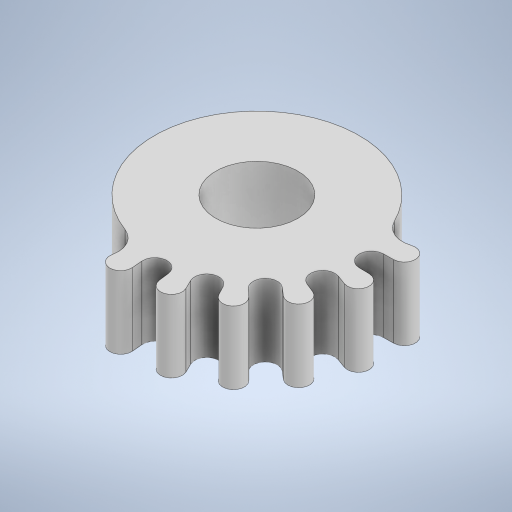
# Autodesk Inventor part: End_Effector_Claw_L_test
Saved by Autodesk Inventor 2023 (Build 270158000, 158)
## iProperties
Created: 2025-02-27
Part Number: End_Effector_Claw_L_test
Material: Generic
Document SubType Name: Modeling
Designer: Swoby
Density: 1 g/cm^3
Appearance: Default
Author: Swoby
Autodesk Inventor part; units mm, degrees
ref_plane "YZ Plane" through (0, 0, 0) normal (1, 0, 0) x (0, 1, 0)
ref_plane "XZ Plane" through (0, 0, 0) normal (0, 1, 0) x (-1, 0, 0)
ref_plane "XY Plane" through (0, 0, 0) normal (0, 0, 1) x (1, 0, 0)
sketch "Sketch1" plane through (0, 0, 0) normal (0, 1, 0) x (-1, 0, 0)
  line L0 (0, 0) -> (10, 0) construction
  circle A0 centre (10, 0) radius 8.5
  line L1 (0, 0) -> (-10, 0) construction
  circle A1 centre (-10, 0) radius 8.5 construction
  line L2 (10, 0) -> (21.547, -20) construction
  line L3 (21.547, -20) -> (21.547, -40) construction
  line L4 (21.547, -40) -> (0, -65.6787) construction
  line L5 (0, -69.6065) -> (0, -61.751)
  arc A2 (0, -61.751) -> (5.0646, -19.2801) centre (-15.4138, -38.3755) ccw
  line L6 (15.5832, -6.4092) -> (26.547, -19.4754) construction
  line L7 (26.547, -19.4754) -> (26.547, -49.4754)
  line L8 (26.547, -49.4754) -> (1.6428, -70.3725)
  arc A3 (4.4168, -6.4092) -> (5.0646, -19.2801) centre (12.3783, -12.4603) ccw
  arc A4 (5.0646, -19.2801) -> (0, -15) centre (-15.4138, -38.3755) ccw construction
  line L9 (15.5832, -6.4092) -> (4.4168, -6.4092) construction
  arc A5 (18.4809, 0.5693) -> (26.547, -19.4754) centre (53.2139, 2.9008) ccw
  arc A6 (0, -69.6065) -> (1.6428, -70.3725) centre (1, -69.6065) ccw
  circle A7 centre (10, 0) radius 1.75
  circle A8 centre (10, 0) radius 3.4
  point P0 (0, -71.751)
  dimension "d0" = 10
  dimension "d1" = 17
  dimension "d2" = 10
  dimension "d3" = 17
  dimension "d4" = 120
  dimension "d5" = 140
  dimension "d6" = 20
  dimension "d9" = 20
  dimension "d10" = 65.6787
  dimension "d11" = 10
  dimension "d12" = 15
  dimension "d14" = 50
  dimension "d15" = 5
  dimension "d16" = 30
  dimension "d18" = 10
  dimension "d19" = 28
  dimension "d20" = 1
  dimension "d52" = 3.5
  dimension "d53" = 6.8
  constraints: 20 end point, 13 point on circle, 9 centre point, 5 tangent, 4 coincident, 4 point on line, 3 horizontal, 3 vertical, 1 midpoint, 1 perpendicular
  measures "d0" distance of L0.start L0.end
  measures "d1" diameter of A0
  measures "d2" distance of L0.start L1.end
  measures "d3" diameter of A1
  measures "d4" angle of L0 L2
  measures "d5" angle of L3 L4
  measures "d6" distance of L2.end L3.end
  measures "d9" vertical distance of L2.start L2.end
  measures "d10" vertical distance of L4.end L0.end
  measures "d11" distance of point (0, -71.751) L5.end
  measures "d12" distance of L0.start A4.end
  measures "d14" angle of L6 L0
  measures "d15" distance between parallel lines of L3 L7
  measures "d16" distance of L6.end L7.end
  measures "d18" radius of A3
  measures "d19" radius of A2
  measures "d20" radius of A6
  measures "d52" diameter of A7
  measures "d53" diameter of A8
extrude "Extrusion1" add sketch "Sketch1" along normal blind 4 contours A0 | A0 A5 L7 L8 A6 L5 A2 A3 | A8
sketch "Sketch2" plane through (0, 4, 0) normal (0, 1, 0) x (1, 0, 0)
  arc A0 (-18.4809, -0.5693) -> (-4.4168, 6.4092) centre (-10, 0) ccw projected
  circle A1 centre (10, 0) radius 8.5 construction
  line L0 (10, 0) -> (18.5, 0) construction
  arc A2 (0.3386, 1.0136) -> (1.2091, 2.0775) centre (0.3242, 1.9135) ccw
  arc A3 (-0.5608, -1.7495) -> (1.2091, -2.0775) centre (0.3242, -1.9135) ccw construction
  circle A4 centre (-0.5, 0) radius 0.9 construction
  line L1 (-10, 0) -> (-18.5, 0) construction
  line L2 (-10, 0) -> (0.3242, 1.9135) construction
  line L3 (-10, 0) -> (0.3242, -1.9135) construction
  arc A5 (-0.516, 0.9999) -> (-0.516, -0.9999) centre (-0.5, 0) ccw
  line L4 (-0.516, 0.9999) -> (0.3386, 1.0136)
  line L5 (-0.516, -0.9999) -> (0.3386, -1.0136)
  arc A6 (-0.5608, 1.7495) -> (0.3386, 1.0136) centre (0.3242, 1.9135) ccw construction
  arc A7 (1.2091, 2.0775) -> (0.0395, 2.7673) centre (0.3242, 1.9135) ccw
  arc A8 (0.3386, -1.0136) -> (-0.5608, -1.7495) centre (0.3242, -1.9135) ccw construction
  arc A9 (1.2091, -2.0775) -> (0.3386, -1.0136) centre (0.3242, -1.9135) ccw
  arc A10 (0.0395, 2.7673) -> (-0.5608, 1.7495) centre (0.3242, 1.9135) ccw construction
  arc A11 (-2.3848, 3.7761) -> (0.0395, 2.7673) centre (-0.593, 4.6646) ccw
  arc A12 (-0.2799, -5.9565) -> (-0.7113, -4.6513) centre (-1.0473, -5.4862) ccw
  line L6 (-1.5043, -4.3322) -> (-0.7113, -4.6513)
  arc A13 (-0.7876, -2.4653) -> (-1.5043, -4.3322) centre (-1.131, -3.4045) ccw
  line L7 (-0.7876, -2.4653) -> (0.0152, -2.7588)
  arc A14 (0.0152, -2.7588) -> (1.2091, -2.0775) centre (0.3242, -1.9135) ccw
  arc A15 (-3.0601, -9.0442) -> (-2.9951, -7.6711) centre (-3.608, -8.3302) ccw
  line L8 (-3.6211, -7.0891) -> (-2.9951, -7.6711)
  arc A16 (-2.283, -5.603) -> (-3.6211, -7.0891) centre (-2.9401, -6.3567) ccw
  line L9 (-2.283, -5.603) -> (-1.6387, -6.1646)
  arc A17 (-1.6387, -6.1646) -> (-0.2799, -5.9565) centre (-1.0473, -5.4862) ccw
  arc A18 (-6.7622, -10.9305) -> (-6.2095, -9.6719) centre (-7.0178, -10.0676) ccw
  line L10 (-6.5853, -8.9042) -> (-6.2095, -9.6719)
  arc A19 (-4.8035, -7.9963) -> (-6.5853, -8.9042) centre (-5.6871, -8.4646) ccw
  line L11 (-4.8035, -7.9963) -> (-4.4033, -8.7516)
  arc A20 (-4.4033, -8.7516) -> (-3.0601, -9.0442) centre (-3.608, -8.3302) ccw
  arc A21 (-10.8944, -11.3649) -> (-9.9274, -10.3879) centre (-10.8238, -10.4676) ccw
  line L12 (-10.0031, -9.5365) -> (-9.9274, -10.3879)
  arc A22 (-8.0143, -9.3275) -> (-10.0031, -9.5365) centre (-9.007, -9.448) ccw
  line L13 (-8.0143, -9.3275) -> (-7.9113, -10.176)
  arc A23 (-7.9113, -10.176) -> (-6.7622, -10.9305) centre (-7.0178, -10.0676) ccw
  arc A24 (-11.7027, -10.2738) -> (-12.9594, -7.9682) centre (-13.6558, -9.843) ccw
  arc A25 (-11.7027, -10.2738) -> (-10.8944, -11.3649) centre (-10.8238, -10.4676) ccw
  point P0 (0, 0)
  point P1 (-9.1115, -8.4534)
  point P2 (-6.1411, -7.5736)
  point P3 (-3.6833, -5.6876)
  point P4 (-2.0646, -3.0461)
  point P5 (-0.2799, -5.9565)
  point P6 (-1.5, 0)
  dimension "d26" = 17
  dimension "d23" = 10
  dimension "d24" = 10
  dimension "d25" = 8.5
  dimension "d36" = 1.8
  dimension "d37" = 1.8
  dimension "d38" = 1.8
  dimension "d39" = 10.5
  dimension "d40" = 10.5
  dimension "d41" = 21
  dimension "d42" = 10.5
  dimension "d43" = 10.5
  dimension "d44" = 2
  dimension "d47" = 84
  dimension "d49" = 2
  dimension "d58" = 9.5
  constraints: 48 point on circle, 28 end point, 24 centre point, 12 tangent, 6 point on line, 2 horizontal, 1 coincident, 1 concentric, 1 horizontal alignment, 59 other
  measures "d23" distance of L1.start point (0, 0)
  measures "d24" distance of L0.start point (0, 0)
  measures "d25" radius of A0
  measures "d36" diameter of A2
  measures "d37" diameter of A3
  measures "d38" diameter of A4
  measures "d39" distance of L1.start L2.end
  measures "d40" distance of L1.start L3.end
  measures "d41" angle of L3 L2
  measures "d42" angle of L1 L2
  measures "d43" distance of L0.start A4.centre
  measures "d44" radius of A11
  measures "d49" radius of A24
  measures "d58" distance of A4.centre L1.start
extrude "Extrusion2" add sketch "Sketch2" against normal up to surface (4 mm away)
extrude "Extrusion4" cut sketch "Sketch1" against normal blind 1 from surface at 4 contours A8
sketch "Sketch3" plane through (0, 4, 0) normal (0, 1, 0) x (1, 0, 0)
  circle A0 centre (-10, 0) radius 3.4 projected
  arc A1 (-4.4168, 6.4092) -> (-5.0646, 19.2801) centre (-12.3783, 12.4603) ccw projected
  arc A2 (0, 61.751) -> (-5.0646, 19.2801) centre (15.4138, 38.3755) ccw projected
  line L0 (0, 61.751) -> (0, 69.6065) projected
  arc A3 (0, 69.6065) -> (-1.6428, 70.3725) centre (-1, 69.6065) ccw projected
  line L1 (-1.6428, 70.3725) -> (-26.547, 49.4754) projected
  line L2 (-26.547, 49.4754) -> (-26.547, 19.4754) projected
  arc A4 (-18.4809, -0.5693) -> (-26.547, 19.4754) centre (-53.2139, -2.9008) ccw projected
  arc A5 (-18.4809, -0.5693) -> (-12.9594, -7.9682) centre (-10, 0) ccw projected
  arc A6 (-11.7027, -10.2738) -> (-12.9594, -7.9682) centre (-13.6558, -9.843) ccw projected
  arc A7 (-11.7027, -10.2738) -> (-9.9274, -10.3879) centre (-10.8238, -10.4676) ccw projected
  line L3 (-9.9274, -10.3879) -> (-10.0031, -9.5365) projected
  arc A8 (-8.0143, -9.3275) -> (-10.0031, -9.5365) centre (-9.007, -9.448) ccw projected
  line L4 (-8.0143, -9.3275) -> (-7.9113, -10.176) projected
  arc A9 (-7.9113, -10.176) -> (-6.2095, -9.6719) centre (-7.0178, -10.0676) ccw projected
  line L5 (-6.2095, -9.6719) -> (-6.5853, -8.9042) projected
  arc A10 (-4.8035, -7.9963) -> (-6.5853, -8.9042) centre (-5.6871, -8.4646) ccw projected
  line L6 (-4.8035, -7.9963) -> (-4.4033, -8.7516) projected
  arc A11 (-4.4033, -8.7516) -> (-2.9951, -7.6711) centre (-3.608, -8.3302) ccw projected
  line L7 (-2.9951, -7.6711) -> (-3.6211, -7.0891) projected
  arc A12 (-2.283, -5.603) -> (-3.6211, -7.0891) centre (-2.9401, -6.3567) ccw projected
  line L8 (-2.283, -5.603) -> (-1.6387, -6.1646) projected
  arc A13 (-1.6387, -6.1646) -> (-0.7113, -4.6513) centre (-1.0473, -5.4862) ccw projected
  line L9 (-0.7113, -4.6513) -> (-1.5043, -4.3322) projected
  arc A14 (-0.7876, -2.4653) -> (-1.5043, -4.3322) centre (-1.131, -3.4045) ccw projected
  line L10 (-0.7876, -2.4653) -> (0.0152, -2.7588) projected
  arc A15 (0.0152, -2.7588) -> (0.3386, -1.0136) centre (0.3242, -1.9135) ccw projected
  line L11 (0.3386, -1.0136) -> (-0.516, -0.9999) projected
  arc A16 (-0.516, 0.9999) -> (-0.516, -0.9999) centre (-0.5, 0) ccw projected
  line L12 (-0.516, 0.9999) -> (0.3386, 1.0136) projected
  arc A17 (0.3386, 1.0136) -> (0.0395, 2.7673) centre (0.3242, 1.9135) ccw projected
  arc A18 (-2.3848, 3.7761) -> (0.0395, 2.7673) centre (-0.593, 4.6646) ccw projected
  arc A19 (-2.3848, 3.7761) -> (-4.4168, 6.4092) centre (-10, 0) ccw projected
  line L13 (-4.4168, 6.4092) -> (-15.6072, 25.7915)
  arc A20 (-15.6072, 25.7915) -> (-26.547, 25.7915) centre (-21.0771, 22.6334) ccw
  line L14 (-26.547, 19.4754) -> (-15.6072, 25.7915) construction
  arc A21 (-26.547, 25.7915) -> (-26.547, 19.4754) centre (-21.0771, 22.6334) ccw construction
  point P0 (0, 0)
  dimension "d59" = 150
  constraints: 4 end point, 4 point on circle, 2 centre point, 2 tangent, 1 perpendicular, 1 point on line
  measures "d59" angle of L13 L2
extrude "Extrusion5" add sketch "Sketch3" along normal blind 2 contours A19 A18 A17 L12 A16 L11 A15 L10 A14 L9 A13 L8 A12 L7 A11 L6 A10 L5 A9 L4 A8 L3 A7 A6 A5 A4 L2 A20 L13
chamfer "Chamfer1" distance 1 angle 45 12 edges at (-12.3892, 0, -41.6909) (-2.3909, 0, -12.9629) (0, 0, -65.6787) (-0.5774, 0, -70.5128) (-14.0949, 0, -59.924) (-26.547, 0, -34.4754) (-12.3892, 4, -41.6909) (-2.3909, 4, -12.9629) (-26.547, 4, -37.6334) (-14.0949, 4, -59.924) (-0.5774, 4, -70.5128) (0, 4, -65.6787)
sketch "Sketch4" plane through (0, 6, 0) normal (0, 1, 0) x (1, 0, 0)
  arc A0 (-15.6072, 25.7915) -> (-26.547, 25.7915) centre (-21.0771, 22.6334) ccw projected
  line L0 (-26.547, 25.7915) -> (-26.547, 19.4754) projected
  arc A1 (-18.4809, -0.5693) -> (-26.547, 19.4754) centre (-53.2139, -2.9008) ccw projected
  arc A2 (-18.4809, -0.5693) -> (-12.9594, -7.9682) centre (-10, 0) ccw projected
  arc A3 (-11.7027, -10.2738) -> (-12.9594, -7.9682) centre (-13.6558, -9.843) ccw projected
  arc A4 (-11.7027, -10.2738) -> (-9.9274, -10.3879) centre (-10.8238, -10.4676) ccw projected
  line L1 (-9.9274, -10.3879) -> (-10.0031, -9.5365) projected
  arc A5 (-8.0143, -9.3275) -> (-10.0031, -9.5365) centre (-9.007, -9.448) ccw projected
  line L2 (-8.0143, -9.3275) -> (-7.9113, -10.176) projected
  arc A6 (-7.9113, -10.176) -> (-6.2095, -9.6719) centre (-7.0178, -10.0676) ccw projected
  line L3 (-6.2095, -9.6719) -> (-6.5853, -8.9042) projected
  arc A7 (-4.8035, -7.9963) -> (-6.5853, -8.9042) centre (-5.6871, -8.4646) ccw projected
  line L4 (-4.8035, -7.9963) -> (-4.4033, -8.7516) projected
  arc A8 (-4.4033, -8.7516) -> (-2.9951, -7.6711) centre (-3.608, -8.3302) ccw projected
  line L5 (-2.9951, -7.6711) -> (-3.6211, -7.0891) projected
  arc A9 (-2.283, -5.603) -> (-3.6211, -7.0891) centre (-2.9401, -6.3567) ccw projected
  line L6 (-2.283, -5.603) -> (-1.6387, -6.1646) projected
  arc A10 (-1.6387, -6.1646) -> (-0.7113, -4.6513) centre (-1.0473, -5.4862) ccw projected
  line L7 (-0.7113, -4.6513) -> (-1.5043, -4.3322) projected
  arc A11 (-0.7876, -2.4653) -> (-1.5043, -4.3322) centre (-1.131, -3.4045) ccw projected
  line L8 (-0.7876, -2.4653) -> (0.0152, -2.7588) projected
  arc A12 (0.0152, -2.7588) -> (0.3386, -1.0136) centre (0.3242, -1.9135) ccw projected
  line L9 (0.3386, -1.0136) -> (-0.516, -0.9999) projected
  arc A13 (-0.516, 0.9999) -> (-0.516, -0.9999) centre (-0.5, 0) ccw projected
  line L10 (-0.516, 0.9999) -> (0.3386, 1.0136) projected
  arc A14 (0.3386, 1.0136) -> (0.0395, 2.7673) centre (0.3242, 1.9135) ccw projected
  arc A15 (-2.3848, 3.7761) -> (0.0395, 2.7673) centre (-0.593, 4.6646) ccw projected
  arc A16 (-2.3848, 3.7761) -> (-4.4168, 6.4092) centre (-10, 0) ccw projected
  line L11 (-4.4168, 6.4092) -> (-15.6072, 25.7915) projected
  circle A17 centre (-10, 0) radius 3.4 projected
  arc A18 (-9.1115, -8.4534) -> (-2.3848, 3.7761) centre (-10, 0) ccw construction
  arc A19 (-12.9594, -7.9682) -> (-9.1115, -8.4534) centre (-10, 0) ccw construction
  arc A20 (-2.3848, 3.7761) -> (-12.9594, -7.9682) centre (-10, 0) ccw
  point P0 (0, 0)
  point P1 (-4.4168, 6.4092)
  point P2 (-18.4809, -0.5693)
  constraints: 9 point on circle, 3 centre point, 1 coincident, 1 concentric
extrude "Extrusion6" cut sketch "Sketch4" against normal through all contours A16 A15 A14 L10 A13 L9 A12 L8 A11 L7 A10 L6 A9 L5 A8 L4 A7 L3 A6 L2 A5 L1 A4 A3 A2 A20 keep common part
equation "\"d3\" = d1"
equation "\"d26\" = 2 * d25"
equation "\"d24\" = d23"
equation "\"d40\" = d39"
equation "\"d42\" = 0.5 * d41"
equation "\"d43\" = d39"
equation "\"d49\" = d44"
body "Solid1"
